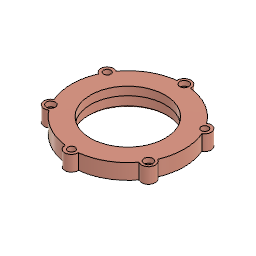
Cover (Autodesk Fusion 360 design; units mm, degrees)
Autodesk Fusion 360 part; units mm, degrees
sketch "Sketch2" plane through (0, 0, 0) normal (0, 0, 1) x (1, 0, 0)
  circle A0 centre (0, 0) radius 34
  circle A1 centre (0, 0) radius 23.5
  circle A2 centre (0, 34) radius 1.65
  circle A3 centre (0, 34) radius 4.15
  circle A4 centre (-29.4449, -17) radius 4.15
  circle A5 centre (-29.4449, -17) radius 1.65
  circle A6 centre (29.4449, -17) radius 4.15
  circle A7 centre (29.4449, -17) radius 1.65
  circle A8 centre (0, 0) radius 31
  circle A9 centre (0, 0) radius 24.5
  circle A10 centre (0, 0) radius 22.5
  circle A11 centre (0, 34) radius 2.7
  circle A12 centre (-29.4449, -17) radius 2.7
  circle A13 centre (29.4449, -17) radius 2.7
  line L0 (0, -34) -> (0, 34) construction
  circle A14 centre (0, -34) radius 2.15
  circle A15 centre (0, -34) radius 3.95
  circle A16 centre (29.4449, 17) radius 3.95
  circle A17 centre (29.4449, 17) radius 2.15
  circle A18 centre (-29.4449, 17) radius 3.95
  circle A19 centre (-29.4449, 17) radius 2.15
  dimension "d19" = 68
  dimension "d21" = 47
  dimension "d22" = 3.3
  dimension "d23" = 2.5
  dimension "d25" = 360
  dimension "d29" = 62
  dimension "d36" = 1
  dimension "d66" = 5.4
  dimension "d68" = 360
  dimension "d83" = 68
  dimension "d84" = 4.3
  dimension "d85" = 1.8
  dimension "d87" = 360
  constraint coincident A0.centre A1.centre
  constraint concentric A0 A1
  constraint coincident A0 A2.centre
  constraint concentric A0 A8
  constraint concentric A2 A11
  constraint vertical L0
  constraint coincident A0 L0.start
  constraint coincident L0.start A14.centre
  measures "d19" diameter of A0
  measures "d21" diameter of A1
  measures "d22" diameter of A2
  measures "d29" diameter of A8
  measures "d66" diameter of A11
  measures "d83" distance of L0.start A2.centre
  measures "d84" diameter of A14
extrude "main" add sketch "Sketch2" along normal blind 5 contours A0 A6 A8 A16 | A0 A8 A16 A17 | A0 A16 A17 | A0 A6 A13 | A0 A6 A8 A13 | A8 A16 | A3 A4 A6 A8 A15 A16 A18 | A0 A7 A13 | A0 A7 A13 | A6 A8 | A0 A3 A8 A16 | A0 A6 A8 A15 | A0 A3 A8 A11 | A3 A8 | A0 A3 A11 | A0 A14 A15 | A0 A8 A14 A15 | A8 A15 | A0 A3 A8 A18 | A0 A2 A11 | A0 A2 A11 | A0 A4 A8 A15 | A8 A18 | A0 A8 A18 A19 | A4 A8 | A0 A4 A8 A12 | A0 A18 A19 | A0 A4 A8 A18 | A0 A4 A12 | A0 A5 A12 | A0 A5 A12 | A1 | A9
extrude "outer ring and heat insert holders" add sketch "Sketch2" against normal blind 4.3 contours A0 A6 A8 A16 | A0 A8 A16 A17 | A0 A16 A17 | A0 A6 A13 | A0 A6 A8 A13 | A0 A7 A13 | A0 A7 A13 | A6 A8 | A0 A3 A8 A16 | A0 A6 A8 A15 | A0 A3 A8 A11 | A3 A8 | A0 A3 A11 | A0 A14 A15 | A0 A8 A14 A15 | A0 A3 A8 A18 | A0 A2 A11 | A0 A2 A11 | A0 A4 A8 A15 | A0 A8 A18 A19 | A4 A8 | A0 A4 A8 A12 | A0 A18 A19 | A0 A4 A8 A18 | A0 A4 A12 | A0 A5 A12 | A0 A5 A12
extrude "bearing mount" add sketch "Sketch2" against normal blind 7 contours A9
extrude "m3 counterbore" cut sketch "Sketch2" against normal blind 4 from surface at 5 contours A0 A7 A13 | A0 A7 A13 | A0 A7 | A0 A7 | A0 A2 A11 | A0 A2 A11 | A0 A2 | A0 A2 | A0 A5 A12 | A0 A5 A12 | A0 A5 | A0 A5
chamfer "Chamfer1" distance 1 angle 45 3 edges at (-31.9621, -16.0236, 1) (26.9276, -16.0236, 1) (-2.5173, 34.9764, 1)
fillet "Fillet3" radius 1 1 edges at (-21.9097, -8.498, -7)
equation "gear_ratio = 6"
equation "gear_Ns = 12"
equation "gear_Nr = ( gear_ratio - 1 ) * gear_Ns"
equation "gear_backlash = 0.25 mm"
equation "gear_OD = ( gear_Nr ) * 1 mm + 8 mm"
equation "thickness = 2 mm"
equation "m3_pilot = 3.3 mm"
equation "d19 = gear_OD"
equation "bearing_od = 47.1 mm"
equation "d21 = bearing_od - bearing_mount_clearance"
equation "d22 = m3_pilot"
equation "d26 = thickness + m3_head_height"
equation "height = 6.5 mm - 2.2 mm"
equation "d29 = gear_OD - wall_thickness"
equation "wall_thickness = 6 mm"
equation "d31 = -height"
equation "bearing_mount_clearance = 0.1 mm"
equation "bearing_width = 7 mm"
equation "bearing_mount_wall_thickness = 1 mm"
equation "d36 = bearing_mount_wall_thickness"
equation "d37 = -bearing_mount_wall_height"
equation "bearing_mount_wall_height = bearing_width"
equation "bearing_mount_lip = 1 mm"
equation "bearing_mount_lip_height = 2 mm"
equation "d46 = -bearing_mount_lip"
equation "m3_inserts = 4.3 mm"
equation "m3_inserts_wall_thickness = 1.8 mm"
equation "m3_head_diameter = 5.2 mm + 0.2 mm"
equation "m3_head_height = 3 mm"
equation "d66 = m3_head_diameter"
equation "d69 = -m3_head_height - m3_chamfer"
equation "m3_chamfer = 1 mm"
equation "d74 = m3_chamfer"
equation "m3_inserts_chamfer = 6.5 mm"
equation "gear_mount_m3_inserts_distance_from_center = 30 mm"
equation "d83 = gear_OD"
equation "d84 = m3_inserts"
equation "d85 = m3_inserts_wall_thickness"
